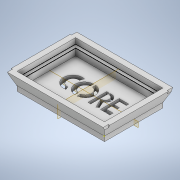
# Autodesk Inventor part: Rack holder Kinpen
Saved by Autodesk Inventor 2021 (Build 250183000, 183)
## iProperties
Created: 2021-05-21
Part Number: Rack holder Kinpen
Material: Generic
Document SubType Name: Modeling
Designer: Olivi
Density: 1 g/cm^3
Appearance: Default
Author: Olivi
Autodesk Inventor part; units mm, degrees
ref_plane "YZ Plane" through (0, 0, 0) normal (1, 0, 0) x (0, 1, 0)
ref_plane "XZ Plane" through (0, 0, 0) normal (0, 1, 0) x (-1, 0, 0)
ref_plane "XY Plane" through (0, 0, 0) normal (0, 0, 1) x (1, 0, 0)
sketch "Sketch1" plane through (0, 0, 0) normal (0, 1, 0) x (-1, 0, 0)
  line L0 (0, 0) -> (0, -85.5)
  line L1 (0, -85.5) -> (127.8, -85.5)
  line L2 (127.8, -85.5) -> (127.8, 0)
  line L3 (127.8, 0) -> (0, 0)
  dimension "d0" = 85.5
  dimension "d1" = 127.8
  constraints: 8 end point, 3 perpendicular, 1 vertical
  measures "d0" distance of L0.start L0.end
  measures "d1" distance of L0.end L1.end
extrude "Extrusion2" add sketch "Sketch1" along normal blind 7
sketch "Sketch3" plane through (0, 7, 0) normal (0, 1, 0) x (1, 0, 0)
  point P0 (0, 0)
sketch "Sketch4" plane through (0, 7, 0) normal (0, 1, 0) x (1, 0, 0)
  arc A0 (-87.0052, 57.9703) -> (-87.3264, 30.9885) centre (-90.5182, 44.5193) ccw
  arc A1 (-88.9325, 52.5097) -> (-88.9325, 35.4855) centre (-89.7687, 43.9976) ccw
  line L0 (-88.9325, 52.5097) -> (-87.0052, 57.9703)
  line L1 (-88.9325, 35.4855) -> (-87.3264, 30.9885)
  arc A2 (-73.8153, 53.315) -> (-74.072, 35.7223) centre (-72.2893, 44.4945) ccw
  arc A3 (-70.5066, 35.7223) -> (-70.7634, 53.315) centre (-72.2893, 44.4945) ccw
  arc A4 (-70.7634, 30.9885) -> (-70.7634, 57.9703) centre (-71.8849, 44.4794) ccw
  line L2 (-70.7634, 57.9703) -> (-70.7634, 53.315)
  line L3 (-70.5066, 35.7223) -> (-70.7634, 30.9885)
  line L4 (-74.072, 35.7223) -> (-74.072, 30.7346)
  line L5 (-73.8153, 57.9703) -> (-73.8153, 53.315)
  arc A5 (-73.8153, 57.9703) -> (-74.072, 30.7346) centre (-73.6823, 44.35) ccw
  line L6 (-54.7714, 57.9703) -> (-54.7714, 30.7346)
  line L7 (-54.7714, 30.7346) -> (-50.7714, 30.7346)
  line L8 (-50.7714, 30.7346) -> (-50.7714, 57.9703)
  line L9 (-50.7714, 57.9703) -> (-54.7714, 57.9703)
  line L10 (-43.1656, 30.7346) -> (-49.5383, 44.3525)
  arc A6 (-49.5383, 44.3525) -> (-49.5383, 55.6427) centre (-48.8397, 49.9976) ccw
  line L11 (-43.1656, 30.7346) -> (-39.7325, 32.3411)
  line L12 (-39.7325, 32.3411) -> (-44.3475, 42.2031)
  arc A7 (-44.3475, 42.2031) -> (-49.5383, 57.9703) centre (-47.7714, 49.814) ccw
  line L13 (-49.5383, 57.9703) -> (-49.5383, 55.6427)
  line L14 (-36.7714, 58.3504) -> (-36.7714, 30.7346)
  line L15 (-36.7714, 30.7346) -> (-22.7714, 30.7346)
  line L16 (-22.7714, 30.7346) -> (-22.7714, 35.5125)
  line L17 (-22.7714, 35.5125) -> (-32.7714, 35.5125)
  line L18 (-32.7714, 35.5125) -> (-32.7714, 43.7637)
  line L19 (-32.7714, 43.7637) -> (-24.9696, 43.7637)
  line L20 (-24.9696, 43.7637) -> (-24.9696, 46.7637)
  line L21 (-24.9696, 46.7637) -> (-32.7714, 46.7637)
  line L22 (-32.7714, 46.7637) -> (-32.7714, 54.7637)
  line L23 (-32.7714, 54.7637) -> (-22.7714, 54.7637)
  line L24 (-22.7714, 54.7637) -> (-22.7714, 58.3504)
  line L25 (-22.7714, 58.3504) -> (-36.7714, 58.3504)
  line L26 (-127.8, 85.5) -> (-127.8, 0) projected
  line L27 (0, 85.5) -> (-127.8, 85.5) projected
  point P0 (0, 0)
  constraints: 52 end point, 19 point on circle, 13 perpendicular, 8 centre point, 6 vertical, 5 point on line, 1 concentric
extrude "Extrusion3" cut sketch "Sketch4" against normal through all
sketch "Sketch5" plane through (0, 7, 0) normal (0, 1, 0) x (1, 0, 0)
  line L0 (-127.8, 0) -> (0, 0) projected
  line L1 (-127.8, 0) -> (0, 0)
  line L2 (0, 0) -> (0, 85.5) projected
  line L3 (0, 0) -> (0, 85.5)
  line L4 (0, 85.5) -> (-127.8, 85.5) projected
  line L5 (0, 85.5) -> (-127.8, 85.5)
  line L6 (-127.8, 85.5) -> (-127.8, 0)
  line L7 (-122.8, 80.5) -> (-5, 80.5)
  line L8 (-5, 80.5) -> (-5, 4.1226)
  line L9 (-5, 4.1226) -> (-122.8, 4.1226)
  line L10 (-122.8, 4.1226) -> (-122.8, 80.5)
  line L11 (-127.8, 85.5) -> (-127.8, 0) projected
  dimension "d44" = 5
  dimension "d45" = 5
  dimension "d46" = 5
  constraints: 16 end point, 5 perpendicular, 3 equal length
  measures "d44" distance between parallel lines of L2 L8
  measures "d45" distance between parallel lines of L6 L10
  measures "d46" distance between parallel lines of L4 L7
extrude "Extrusion4" add sketch "Sketch5" along normal blind 10
sketch "Sketch9" plane through (0, 17, 0) normal (0, 1, 0) x (1, 0, 0)
  line L0 (-127.8, 85.5) -> (-127.8, 0) projected
  line L1 (-127.8, 0) -> (-127.8, 85.5)
  line L2 (-127.8, 85.5) -> (0, 85.5)
  line L3 (0, 85.5) -> (0, 0)
  line L4 (0, 0) -> (-127.8, 0)
  line L5 (-122.8, 4.1226) -> (-5, 4.1226) projected
  line L6 (-5, 80.5) -> (-122.8, 80.5) projected
  line L7 (-122.8, 4.1226) -> (-122.8, 80.5)
  line L8 (-122.8, 80.5) -> (-5, 80.5)
  line L9 (-5, 80.5) -> (-5, 4.1226)
  line L10 (-5, 4.1226) -> (-122.8, 4.1226)
  point P0 (0, 0)
  constraints: 16 end point, 5 equal length, 3 perpendicular
ref_plane "Work Plane4" through (-63.9, 0, 0) normal (1, 0, 0) x (0, 0, -1)
sketch "Sketch21" plane through (-63.9, 0, 0) normal (1, 0, 0) x (0, 0, -1)
  line L0 (0, 0) -> (0, 17) projected
  line L1 (0, 7.0438) -> (0, 25.0438)
  line L2 (0, 25.0438) -> (-8, 25.0438)
  line L3 (-8, 25.0438) -> (0, 7.0438)
  line L4 (85.5, 0) -> (85.5, 17) projected
  line L5 (85.5, 7.0438) -> (85.5, 25.0438)
  line L6 (85.5, 25.0438) -> (93.5, 25.0438)
  line L7 (93.5, 25.0438) -> (85.5, 7.0438)
  dimension "d99" = 18
  dimension "d100" = 8
  dimension "d101" = 18
  dimension "d102" = 8
  constraints: 12 end point, 2 collinear, 2 perpendicular, 2 point on line
  measures "d99" distance of L1.start L1.end
  measures "d100" distance of L1.end L2.end
  measures "d101" distance of L5.start L5.end
  measures "d102" distance of L5.end L6.end
extrude "Extrusion7" add sketch "Sketch21" along normal mid plane 140
ref_plane "Work Plane5" through (-127.8, 0, -42.7) normal (0, 0, 1) x (1, 0, 0)
sketch "Sketch22" plane through (-127.8, 0, -42.7) normal (0, 0, 1) x (1, 0, 0)
  line L0 (127.8, 7.0438) -> (133.9, 7.0438) projected
  line L1 (127.8, 7.0438) -> (127.8, 25.0438)
  line L2 (133.9, 25.0438) -> (-6.1, 25.0438) projected
  line L3 (127.8, 25.0438) -> (135.8, 25.0438)
  line L4 (135.8, 25.0438) -> (127.8, 7.0438)
  line L5 (0, 0) -> (0, 7.0438) projected
  line L6 (0, 7.0438) -> (0, 25.0438)
  line L7 (0, 25.0438) -> (-8, 25.0438)
  line L8 (-6.1, 7.0438) -> (0, 7.0438) projected
  line L9 (-8, 25.0438) -> (0, 7.0438)
  point P0 (127.8, 0)
  dimension "d106" = 8
  dimension "d107" = 8
  constraints: 12 end point, 3 point on line, 2 perpendicular, 1 vertical
  measures "d106" distance of L1.end L3.end
  measures "d107" distance of L6.end L7.end
extrude "Extrusion8" add sketch "Sketch22" along normal mid plane 86
sketch "Sketch24" plane through (-127.8, 0, 0) normal (0, 0, 1) x (1, 0, 0)
  line L0 (-6.1, 7.0438) -> (-6.1, 25.0438) projected
  line L1 (0, 7.0438) -> (127.8, 7.0438) projected
  line L2 (-6.1, 20.9849) -> (0, 7.0438)
  line L3 (0, 7.0438) -> (-6.1, 7.0438)
  line L4 (-6.1, 7.0438) -> (-6.1, 20.9849)
  line L5 (127.8, 7.0438) -> (133.9, 7.0438) projected
  line L6 (133.9, 7.0438) -> (133.9, 20.7688) projected
  line L7 (127.8, 7.0438) -> (133.9, 20.7688)
  line L8 (133.9, 20.7688) -> (133.9, 7.0438)
  line L9 (133.9, 7.0438) -> (127.8, 7.0438)
  point P0 (127.8, 0)
  constraints: 12 end point, 2 collinear, 2 perpendicular, 1 point on line
extrude "Extrusion9" cut sketch "Sketch24" along normal blind 86
sketch "Sketch25" plane through (0, 0, -85.5) normal (0, 0, -1) x (-1, 0, 0)
  line L0 (-6.1, 20.7688) -> (0, 7.0438) projected
  line L1 (0, 7.0438) -> (-6.1, 20.7688)
  line L2 (-6.1, 20.7688) -> (-6.1, 7.0438)
  line L3 (-6.1, 7.0438) -> (0, 7.0438)
  line L4 (127.8, 7.0438) -> (133.9, 20.7688) projected
  line L5 (127.8, 7.0438) -> (133.9, 20.7688)
  line L6 (133.9, 7.0438) -> (133.9, 20.7688) projected
  line L7 (133.9, 20.7688) -> (133.9, 7.0438)
  line L8 (127.8, 7.0438) -> (0, 7.0438) projected
  line L9 (133.9, 7.0438) -> (127.8, 7.0438)
  point P0 (0, 0)
  constraints: 12 end point, 3 collinear, 2 perpendicular, 1 point on line, 1 vertical
extrude "Extrusion10" cut sketch "Sketch25" along normal blind 86
body "Solid2"
